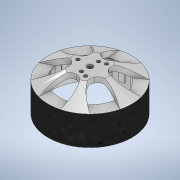
# Autodesk Inventor part: Rotor2
Saved by Autodesk Inventor 2020.2 (Build 242310000, 310)
## iProperties
Created: 2020-02-19
Part Number: Rotor2
Material: Aluminum 6061-AHC
Document SubType Name: Modeling
Designer: user
Density: 2.7 g/cm^3
Appearance: Aluminum - Dark
Mass: 37.7891 g
Surface Area: 122.177 cm^2
Volume: 13.996 cm^3
Author: user
Autodesk Inventor part; units mm, degrees
ref_plane "YZ Plane" through (0, 0, 0) normal (1, 0, 0) x (0, 1, 0)
ref_plane "XZ Plane" through (0, 0, 0) normal (0, 1, 0) x (-1, 0, 0)
sketch "Sketch1" plane through (0, 0, 0) normal (0, 0, 1) x (1, 0, 0)
  line L0 (0, 0) -> (0, 33.5)
  line L1 (0, 33.5) -> (12.5, 33.5)
  line L2 (12.5, 33.5) -> (29.5, 25.3218)
  line L3 (29.5, 25.3218) -> (29.5, 4.8218)
  line L4 (0, 33.5) -> (0, 30)
  line L5 (0, 30) -> (11.7019, 30)
  line L6 (11.7019, 30) -> (27, 22.6406)
  line L7 (27, 22.6406) -> (27, 5.5283)
  line L8 (27, 5.5283) -> (29.5, 4.8218)
  point P0 (22.5, 0)
  dimension "d0" = 33.5
  dimension "d1" = 59
  dimension "d2" = 20.5
  dimension "d3" = 25
  dimension "d6" = 3.5
  dimension "d7" = 3.5
  constraints: 18 end point, 5 coincident, 2 parallel, 2 perpendicular, 1 horizontal, 1 point on line, 1 vertical
  measures "d0" distance of L0.start L0.end
  measures "d1" diameter of L3 L0
  measures "d2" distance of L2.end L3.end
  measures "d3" diameter of L1.end L0
  measures "d6" distance between parallel lines of L5 L1
  measures "d7" distance between parallel lines of L6 L2
revolve "Revolution1" add sketch "Sketch1" angle 360 about axis through (0, 0, 0) along (0, 1, 0)
sketch "Sketch2" plane through (0, 33.5, 0) normal (0, 1, 0) x (1, 0, 0)
  circle A0 centre (0, 0) radius 29.5 projected
  circle A1 centre (0, 0) radius 29.5 projected
  line L0 (-7.75, 28.4638) -> (7.75, 28.4638)
  line L1 (0, 0) -> (0, 29.5)
  line L2 (-7.75, 28.4638) -> (-7.75, 9.5) construction
  line L3 (-7.75, 9.5) -> (0, 9.5) construction
  spline S0 degree 2 poles (-7.75, 28.4638) (-7.75, 9.5) (0, 9.5) knots 1 1 1 2 2 2
  line L4 (7.75, 28.4638) -> (7.75, 9.5) construction
  line L5 (7.75, 9.5) -> (0, 9.5) construction
  spline S1 degree 2 poles (7.75, 28.4638) (7.75, 9.5) (0, 9.5) knots 1 1 1 2 2 2
  dimension "d12" = 15.5
  dimension "d19" = 20
  constraints: 4 end point, 3 point on circle, 2 perpendicular, 1 horizontal, 1 point on line, 1 symmetric about line, 1 vertical, 6 other
  measures "d12" distance of L0.start L0.end
  measures "d19" distance of L3.end L1.end
sketch3d "3D Sketch1"
ref_plane "Work Plane1" through (28.129, 25.3218, 8.8886) normal (0, 1, 0) x (1, 0, 0)
extrude "Extrusion1" cut sketch "Sketch2" against normal up to surface (8.1782 mm away) contours L0 L1 A0 | S1 L1 L0 | A0 L1 L0 | L0 L1 S0
pattern_circular "Circular Pattern1" count 6 over 360 about axis through (0, -10, 0) along (0, 1, 0) of "Extrusion1"
sketch "Sketch3" plane through (0, 33.5, 0) normal (0, 1, 0) x (1, 0, 0)
  arc A0 (7.9451, 9.6502) -> (4.3848, 11.7057) centre (0, 0) ccw projected
  arc A1 (-4.3848, 11.7057) -> (-7.9451, 9.6502) centre (0, 0) ccw projected
  arc A2 (-12.3298, 2.0555) -> (-12.3298, -2.0555) centre (0, 0) ccw projected
  arc A3 (-7.9451, -9.6502) -> (-4.3848, -11.7057) centre (0, 0) ccw projected
  arc A4 (4.3848, -11.7057) -> (7.9451, -9.6502) centre (0, 0) ccw projected
  arc A5 (12.3298, -2.0555) -> (12.3298, 2.0555) centre (0, 0) ccw projected
  constraints: 12 other
sketch "Sketch4" plane through (0, 33.5, 0) normal (0, 1, 0) x (1, 0, 0)
  arc A0 (7.9451, 9.6502) -> (4.3848, 11.7057) centre (0, 0) ccw projected
  arc A1 (-12.3298, 2.0555) -> (-12.3298, -2.0555) centre (0, 0) ccw projected
  arc A2 (12.3298, -2.0555) -> (12.3298, 2.0555) centre (0, 0) ccw projected
  arc A3 (-13.8247, 16.3698) -> (-21.089, 3.7876) centre (0, 0) ccw projected
  circle A4 centre (0, 0) radius 8.5
  line L0 (-12.5, 0) -> (12.5, 0)
  point P0 (0, 6)
  point P1 (0, -6)
  point P2 (-8.5, 0)
  point P3 (4.25, -7.3612)
  point P4 (4.25, 7.3612)
  dimension "d20" = 17
  dimension "d21" = 12
  dimension "d24" = 360
  constraints: 2 end point, 2 point on circle, 1 coincident, 1 horizontal alignment, 1 point on line, 1 symmetric about line, 6 other
  measures "d21" distance of point (0, -6) point (0, 6)
hole "Hole1" at (-8.5, 33.5, 0) at (4.25, 33.5, -7.3612) at (0, 33.5, 6) at (0, 33.5, -6) at (4.25, 33.5, 7.3612) direction (0, -1, 0) diameter 2.459 end through all thread size "M3x0.5" class "6H" standard "ANSI Metric M Profile"
sketch "Sketch5" plane through (0, 33.5, 0) normal (0, 1, 0) x (1, 0, 0)
  arc A0 (12.3298, -2.0555) -> (12.3298, 2.0555) centre (0, 0) ccw projected
  circle A1 centre (0, 0) radius 2
  dimension "d33" = 4
  constraints: 1 centre point, 1 coincident
  measures "d33" diameter of A1
extrude "Extrusion2" cut sketch "Sketch5" against normal through all
ref_plane "Work Plane2" through (28.129, 21.0718, 8.8886) normal (0, 1, 0) x (1, 0, 0)
sketch "Sketch6" plane through (28.129, 21.0718, 8.8886) normal (0, 1, 0) x (1, 0, 0)
  circle A0 centre (-28.129, 8.8886) radius 27 projected
  circle A1 centre (-28.129, 8.8886) radius 15
  arc A2 (-2.1462, 12.6244) -> (-1.9285, 10.499) centre (-28.129, 8.8886) ccw
  line L0 (-1.879, 8.8886) -> (-1.129, 8.8886)
  line L1 (-2.1462, 12.6244) -> (-1.4039, 12.7311)
  line L2 (-2.9423, 16.2841) -> (-2.2227, 16.4954)
  line L3 (-4.2512, 19.7933) -> (-3.569, 20.1048)
  line L4 (-6.0461, 23.0804) -> (-5.4152, 23.4859)
  line L5 (-8.2906, 26.0787) -> (-7.7238, 26.5699)
  line L6 (-10.9389, 28.727) -> (-10.4478, 29.2939)
  line L7 (-13.9372, 30.9715) -> (-13.5317, 31.6025)
  line L8 (-17.2244, 32.7665) -> (-16.9128, 33.4487)
  line L9 (-20.7336, 34.0753) -> (-20.5223, 34.7949)
  line L10 (-24.3933, 34.8714) -> (-24.2865, 35.6138)
  line L11 (-28.129, 35.1386) -> (-28.129, 35.8886)
  line L12 (-31.8648, 34.8714) -> (-31.9715, 35.6138)
  line L13 (-35.5245, 34.0753) -> (-35.7358, 34.7949)
  line L14 (-39.0337, 32.7665) -> (-39.3452, 33.4487)
  line L15 (-42.3209, 30.9715) -> (-42.7263, 31.6025)
  line L16 (-45.3191, 28.727) -> (-45.8103, 29.2939)
  line L17 (-47.9675, 26.0787) -> (-48.5343, 26.5699)
  line L18 (-50.2119, 23.0804) -> (-50.8429, 23.4859)
  line L19 (-52.0069, 19.7933) -> (-52.6891, 20.1048)
  line L20 (-53.3157, 16.2841) -> (-54.0353, 16.4954)
  line L21 (-54.1118, 12.6244) -> (-54.8542, 12.7311)
  line L22 (-54.379, 8.8886) -> (-55.129, 8.8886)
  line L23 (-54.1118, 5.1529) -> (-54.8542, 5.0461)
  line L24 (-53.3157, 1.4931) -> (-54.0353, 1.2818)
  line L25 (-52.0069, -2.016) -> (-52.6891, -2.3276)
  line L26 (-50.2119, -5.3032) -> (-50.8429, -5.7087)
  line L27 (-47.9675, -8.3015) -> (-48.5343, -8.7926)
  line L28 (-45.3191, -10.9498) -> (-45.8103, -11.5166)
  line L29 (-42.3209, -13.1943) -> (-42.7263, -13.8252)
  line L30 (-39.0337, -14.9892) -> (-39.3452, -15.6714)
  line L31 (-35.5245, -16.2981) -> (-35.7358, -17.0177)
  line L32 (-31.8648, -17.0942) -> (-31.9715, -17.8366)
  line L33 (-28.129, -17.3614) -> (-28.129, -18.1114)
  line L34 (-24.3933, -17.0942) -> (-24.2865, -17.8366)
  line L35 (-20.7336, -16.2981) -> (-20.5223, -17.0177)
  line L36 (-17.2244, -14.9892) -> (-16.9128, -15.6714)
  line L37 (-13.9372, -13.1943) -> (-13.5317, -13.8252)
  line L38 (-10.9389, -10.9498) -> (-10.4478, -11.5166)
  line L39 (-8.2906, -8.3015) -> (-7.7238, -8.7926)
  line L40 (-6.0461, -5.3032) -> (-5.4152, -5.7087)
  line L41 (-4.2512, -2.016) -> (-3.569, -2.3276)
  line L42 (-2.9423, 1.4931) -> (-2.2227, 1.2818)
  line L43 (-2.1462, 5.1529) -> (-1.4039, 5.0461)
  line L44 (-1.879, 8.8886) -> (-13.129, 8.8886)
  line L45 (-1.9285, 7.2782) -> (-1.1837, 7.1711)
  arc A3 (-1.9285, 10.499) -> (-2.1462, 12.6244) centre (-28.129, 8.8886) ccw
  line L46 (-1.9285, 10.499) -> (-1.1837, 10.6061)
  dimension "d37" = 30
  dimension "d38" = 52.5
  dimension "d41" = 360
  constraints: 94 end point, 9 point on circle, 2 centre point, 2 coincident, 2 horizontal, 1 horizontal alignment, 1 parallel, 135 other
  measures "d38" diameter of A2
extrude "Extrusion3" add sketch "Sketch6" against normal blind 12 contours L0 A2 L46 A0 | A0 L45 A2 L0
pattern_circular "Circular Pattern2" count 22 over 360 about axis through (0, -10, 0) along (0, 1, 0) of "Extrusion3"
equation "\"d7\" = d6"
body "Solid1"
